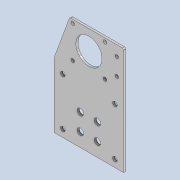
# Autodesk Inventor part: X Axis Belt Motor Frame Machined
Saved by Autodesk Inventor 2022 (Build 260153000, 153)
## iProperties
Created: 2021-10-17
Part Number: X Axis Belt Motor Frame Machined
Material: Generic
Document SubType Name: Modeling
Designer: Coy
Density: 1 g/cm^3
Appearance: Machined - Aluminum
Author: Coy
Autodesk Inventor part; units mm, degrees
ref_plane "YZ Plane" through (0, 0, 0) normal (1, 0, 0) x (0, 1, 0)
ref_plane "XZ Plane" through (0, 0, 0) normal (0, 1, 0) x (-1, 0, 0)
ref_plane "XY Plane" through (0, 0, 0) normal (0, 0, 1) x (1, 0, 0)
sketch "Sketch1" plane through (0, 0, 0) normal (0, 0, 1) x (1, 0, 0)
  line L0 (-88.9, 80.5892) -> (-12.7, 80.5892) construction
  line L1 (-12.7, 80.5892) -> (-12.7, 10.7392) construction
  line L2 (-12.7, 10.7392) -> (-88.9, 10.7392) construction
  line L3 (-88.9, 10.7392) -> (-88.9, 80.5892) construction
  line L4 (-88.9, 80.5892) -> (-88.9, 97.6783) construction
  line L5 (-88.9, 80.5892) -> (-101.6, 80.5892) construction
  line L6 (-101.6, 95.25) -> (-101.6, -6.35)
  line L7 (-12.7, 10.7392) -> (-12.7, -6.35) construction
  line L8 (0, -6.35) -> (-101.6, -6.35)
  line L9 (-12.7, 10.7392) -> (0, 10.7392) construction
  line L10 (0, 95.25) -> (0, -6.35)
  circle A0 centre (-12.7, 80.5892) radius 3.325
  circle A1 centre (-12.7, 10.7392) radius 3.325
  circle A2 centre (-88.9, 10.7392) radius 3.325
  circle A3 centre (-88.9, 80.5892) radius 3.325
  circle A4 centre (-63.3, 45.15) radius 2.1 construction
  circle A5 centre (-63.3, 20.15) radius 2.1 construction
  circle A6 centre (-38.3, 45.15) radius 2.1 construction
  circle A7 centre (-38.3, 20.15) radius 2.1 construction
  circle A8 centre (-63.3, 45.15) radius 4.7625
  circle A9 centre (-38.3, 45.15) radius 2.1 construction
  circle A10 centre (-38.3, 45.15) radius 4.7625
  circle A11 centre (-63.3, 20.15) radius 2.1 construction
  circle A12 centre (-63.3, 20.15) radius 4.7625
  circle A13 centre (-38.3, 20.15) radius 2.1 construction
  circle A14 centre (-38.3, 20.15) radius 4.7625
  line L11 (0, 95.25) -> (-101.6, 95.25) construction
  line L12 (-22.6, 156.65) -> (-79, 156.65) construction
  line L13 (-79, 156.65) -> (-79, 100.25) construction
  line L14 (-79, 100.25) -> (-22.6, 100.25) construction
  line L15 (-22.6, 100.25) -> (-22.6, 156.65) construction
  line L16 (-22.6, 128.45) -> (-79, 128.45) construction
  line L17 (-113.7839, 128.45) -> (12.1839, 128.45) construction
  line L18 (-27.23, 152.02) -> (-74.37, 152.02) construction
  line L19 (-74.37, 152.02) -> (-74.37, 104.88) construction
  line L20 (-74.37, 104.88) -> (-27.23, 104.88) construction
  line L21 (-27.23, 104.88) -> (-27.23, 152.02) construction
  line L22 (-27.23, 152.02) -> (-22.6, 152.02) construction
  line L23 (-27.23, 152.02) -> (-27.23, 156.65) construction
  line L24 (-74.37, 104.88) -> (-79, 104.88) construction
  line L25 (-74.37, 104.88) -> (-74.37, 100.25) construction
  circle A15 centre (-27.23, 152.02) radius 2.6
  circle A16 centre (-27.23, 104.88) radius 2.6
  circle A17 centre (-74.37, 104.88) radius 2.6
  circle A18 centre (-74.37, 152.02) radius 2.6
  circle A19 centre (-50.8, 128.45) radius 19.15
  circle A20 centre (-50.8, 128.45) radius 11.08 construction
  circle A21 centre (-50.8, 128.45) radius 13 construction
  line L26 (-50.8, -6.35) -> (-50.8, 203.8417) construction
  circle A22 centre (-74.37, 104.88) radius 13 construction
  circle A23 centre (-27.23, 104.88) radius 13 construction
  circle A24 centre (-74.37, 104.88) radius 11.08 construction
  circle A25 centre (-27.23, 104.88) radius 11.08 construction
  line L27 (-79, 157.1) -> (-101.6, 95.25)
  line L28 (0, 95.25) -> (-22.6, 157.1)
  line L29 (0, 0) -> (-101.6, 0)
  line L30 (-79, 157.1) -> (-22.6, 157.1)
  line L31 (-63.3, 45.15) -> (-38.3, 45.15) construction
  line L32 (-38.3, 45.15) -> (-38.3, 20.15) construction
  line L33 (-38.3, 20.15) -> (-63.3, 20.15) construction
  line L34 (-63.3, 20.15) -> (-63.3, 45.15) construction
  line L35 (0, 95.25) -> (0, 157.1)
  line L36 (0, 157.1) -> (-22.6, 157.1)
  point P0 (-39.7703, 127.3952)
  point P1 (-39.7703, 127.3951)
  point P2 (-50.8, 128.45)
  dimension "d0" = 6.65
  dimension "d1" = 6.65
  dimension "d2" = 6.65
  dimension "d3" = 6.65
  dimension "d4" = 69.85
  dimension "d5" = 76.2
  dimension "d6" = 9.525
  dimension "d7" = 9.525
  dimension "d8" = 9.525
  dimension "d9" = 9.525
  dimension "d10" = 101.6
  dimension "d12" = 56.4
  dimension "d13" = 56.4
  dimension "d14" = 0
  dimension "d15" = 47.14
  dimension "d16" = 47.14
  dimension "d17" = 5.2
  dimension "d18" = 5.2
  dimension "d19" = 5.2
  dimension "d20" = 5.2
  dimension "d21" = 38.3
  dimension "d22" = 22.16
  dimension "d23" = 26
  dimension "d24" = 28.2
  dimension "d25" = 50.8
  dimension "d26" = 5
  dimension "d27" = 95.25
  dimension "d28" = 26
  dimension "d29" = 26
  dimension "d30" = 22.16
  dimension "d31" = 22.16
  dimension "d34" = 0.45
  dimension "d36" = 25
  dimension "d37" = 25
  dimension "d38" = 26.5
  constraints: 74 end point, 26 centre point, 23 coincident, 12 parallel, 10 perpendicular, 9 point on line, 8 horizontal, 5 midpoint, 4 vertical, 2 point on circle
  measures "d0" diameter of A0
  measures "d1" diameter of A1
  measures "d2" diameter of A2
  measures "d3" diameter of A3
  measures "d4" distance of L2.end L0.start
  measures "d5" distance of L0.start L0.end
  measures "d6" diameter of A8
  measures "d7" diameter of A10
  measures "d8" diameter of A12
  measures "d9" diameter of A14
  measures "d10" distance between parallel lines of L11 L8
  measures "d12" distance of L15.start L13.end
  measures "d13" distance of L13.start L13.end
  measures "d14" distance between parallel lines of L17 L16
  measures "d15" distance of L21.start L21.end
  measures "d16" distance of L19.end L21.start
  measures "d17" diameter of A15
  measures "d18" diameter of A16
  measures "d19" diameter of A17
  measures "d20" diameter of A18
  measures "d21" diameter of A19
  measures "d22" diameter of A20
  measures "d23" diameter of A21
  measures "d24" distance from line of L15 A21.centre
  measures "d25" distance from line of L29.start L26
  measures "d26" distance between parallel lines of L11 L14
  measures "d27" distance from line of L29.start L11
  measures "d28" diameter of A22
  measures "d29" diameter of A23
  measures "d30" diameter of A24
  measures "d31" diameter of A25
  measures "d34" distance between parallel lines of L12 L30
  measures "d36" distance of L31.start L31.end
  measures "d37" distance of L33.end L31.start
  measures "d38" distance between parallel lines of L8 L33
extrude "Extrusion1" add sketch "Sketch1" against normal blind 3.175 contours L27 L30 L28 L10 L29 L6 | L36 L35 L28
fillet "Fillet1" radius 2 3 edges at (-79, 157.1, -1.5875) (-101.6, 95.25, -1.5875) (0, 157.1, -1.5875)
sketch "Sketch2" plane through (0, 0, -3.175) normal (0, 0, -1) x (-1, 0, 0)
  line L0 (0, 157.1) -> (20, 157.1) construction
  line L1 (20, 157.1) -> (20, 102.1) construction
  line L2 (20, 102.1) -> (0, 102.1) construction
  line L3 (0, 102.1) -> (0, 157.1) construction
  line L4 (77.6015, 157.1) -> (2, 157.1) construction
  line L5 (0, 155.1) -> (0, 0) construction
  line L6 (10, 102.1) -> (10, 157.1) construction
  line L7 (2, 157.1) -> (77.6015, 157.1) construction
  circle A0 centre (10, 142.1) radius 2.6
  circle A1 centre (10, 117.1) radius 2.6
  dimension "d39" = 20
  dimension "d40" = 55
  dimension "d41" = 5.2
  dimension "d42" = 5.2
  dimension "d43" = 15
  dimension "d44" = 15
  constraints: 10 end point, 3 point on line, 2 centre point, 2 collinear, 2 parallel, 2 perpendicular, 1 horizontal, 1 midpoint
  measures "d39" distance of L1.end L2.end
  measures "d40" distance of L0.end L1.end
  measures "d41" diameter of A0
  measures "d42" diameter of A1
  measures "d43" distance from line of L0 A0.centre
  measures "d44" distance of L6.start A1.centre
extrude "Extrusion2" cut sketch "Sketch2" against normal up to next
equation "\"d0\" = d3"
equation "\"d1\" = d3"
equation "\"d2\" = d3"
equation "\"d7\" = d6"
equation "\"d8\" = d6"
equation "\"d9\" = d6"
equation "\"d16\" = d15"
equation "\"d18\" = d17"
equation "\"d19\" = d17"
equation "\"d20\" = d17"
equation "\"d24\" = 0.5 * d12"
equation "\"d44\" = d43"
body "Solid1"
